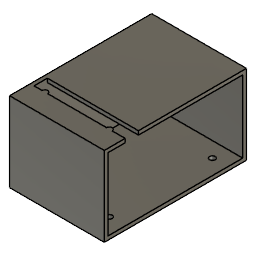
Tic housing (Autodesk Fusion 360 design; units mm, degrees)
Autodesk Fusion 360 part; units mm, degrees
sketch "Sketch1" plane through (0, 0, 0) normal (0, 0, 1) x (1, 0, 0)
  line L0 (-25, 50) -> (25, 50)
  line L1 (25, 50) -> (25, -25)
  line L2 (25, -25) -> (-25, -25)
  line L3 (-25, -25) -> (-25, 50)
  circle A0 centre (-17.3027, -14) radius 1.5
  circle A1 centre (16.6973, -14) radius 1.5
  circle A2 centre (-17, 40) radius 1.5
  circle A3 centre (17, 39.9992) radius 1.5
  dimension "d1" = 3
  dimension "d2" = 3
  dimension "d4" = 34
  dimension "d5" = 3
  dimension "d6" = 54
  dimension "d7" = 3
  dimension "d9" = 34
  dimension "d10" = 54
  constraint horizontal L0
  constraint vertical L1
  constraint horizontal L2
  constraint vertical L3
  measures "d1" diameter of A0
  measures "d2" diameter of A1
  measures "d4" horizontal distance of A0.centre A1.centre
  measures "d5" diameter of A2
  measures "d6" vertical distance of A0.centre A2.centre
  measures "d7" diameter of A3
  measures "d9" horizontal distance of A2.centre A3.centre
  measures "d10" distance of A1.centre A3.centre
extrude "Extrude1" add sketch "Sketch1" along normal blind 2 makes body 1
ref_plane "WorkPlane1" through (0, 12.5, 3) normal (0, 0, 1) x (1, 0, 0)
ref_plane "WorkPlane2" through (0, 12.5, 42) normal (0, 0, 1) x (1, 0, 0)
sketch "Sketch4" plane through (0, 0, 42) normal (0, 0, 1) x (1, 0, 0)
sketch "Sketch5" plane through (0, 0, 42) normal (0, 0, 1) x (1, 0, 0)
  line L0 (25, -25) -> (-25, -25)
  line L1 (-25, -25) -> (-25, 50)
  line L2 (-25, 50) -> (25, 50)
  line L3 (25, 50) -> (25, -25)
  constraint horizontal L0
  constraint vertical L1
  constraint horizontal L2
  constraint vertical L3
extrude "Extrude2" add sketch "Sketch5" against normal blind 2 separate body makes body 2
sketch "Sketch6" plane through (0, 0, 2) normal (0, 0, 1) x (-1, 0, 0)
  circle A0 centre (17, -40) radius 1.5
  circle A1 centre (-16.6973, 14) radius 1.5
  circle A2 centre (-17, -39.9992) radius 1.5
  circle A3 centre (17.3027, 14) radius 1.5
  line L0 (25, 25) -> (-25, 25)
  line L1 (-25, 25) -> (-25, -50)
  line L2 (-25, -50) -> (25, -50)
  line L3 (25, -50) -> (25, 25)
  line L4 (25, -50) -> (23, -50)
  line L5 (23, -50) -> (23, 25)
  line L6 (23, 25) -> (25, 25)
  line L7 (25, 25) -> (25, -50)
  constraint horizontal L4
  constraint vertical L5
  constraint horizontal L6
  constraint vertical L7
  constraint coincident L0 L5.end
  constraint coincident L2.end L3.start
extrude "Extrude3" add sketch "Sketch6" along normal blind 39 contours L0 L2 L3 L4 L5 L6 L7 bodies 1 2
sketch "Sketch7" plane through (0, 0, 2) normal (0, 0, 1) x (-1, 0, 0)
  line L0 (23, -50) -> (23, 25)
  line L1 (23, 25) -> (-25, 25)
  line L2 (-25, 25) -> (-25, -50)
  line L3 (-25, -50) -> (23, -50)
  circle A0 centre (17.3027, 14) radius 1.5
  circle A1 centre (-17, -39.9992) radius 1.5
  circle A2 centre (-16.6973, 14) radius 1.5
  circle A3 centre (17, -40) radius 1.5
  line L4 (23, 25) -> (-25, 25)
  line L5 (-25, 25) -> (-25, 23)
  line L6 (-25, 23) -> (23, 23)
  line L7 (23, 23) -> (23, 25)
  line L8 (23, -50) -> (-25, -50)
  line L9 (-25, -50) -> (-25, -48)
  line L10 (-25, -48) -> (23, -48)
  line L11 (23, -48) -> (23, -50)
  constraint horizontal L4
  constraint vertical L5
  constraint horizontal L6
  constraint vertical L7
  constraint coincident L2 L5.end
  constraint coincident L0.end L1.start
  constraint horizontal L8
  constraint vertical L9
  constraint horizontal L10
  constraint vertical L11
  constraint coincident L2 L9.end
  constraint coincident L0.start L3.end
extrude "Extrude4" add sketch "Sketch7" along normal blind 38 contours L0 L2 L3 L8 L9 L10 L11 bodies 1
extrude "Extrude5" add sketch "Sketch7" along normal blind 38 contours L0 L1 L2 L4 L5 L6 L7 bodies 1
sketch "Sketch8" plane through (0, 0, 2) normal (0, 0, 1) x (-1, 0, 0)
  line L0 (23, 23) -> (-25, 23)
  line L1 (-25, 23) -> (-25, -48)
  line L2 (-25, -48) -> (23, -48)
  line L3 (23, -48) -> (23, 23)
  circle A0 centre (17, -40) radius 1.5
  circle A1 centre (-16.6973, 14) radius 1.5
  circle A2 centre (-17, -39.9992) radius 1.5
  circle A3 centre (17.3027, 14) radius 1.5
  line L4 (23, 14) -> (-25, 14)
  line L5 (-25, 14) -> (-25, 7)
  line L6 (-25, 7) -> (23, 7)
  line L7 (23, 7) -> (23, 14)
  constraint horizontal L4
  constraint vertical L5
  constraint horizontal L6
  constraint vertical L7
  constraint coincident L1 L5.end
  constraint coincident L3 L4.start
extrude "Extrude6" cut sketch "Sketch8" along normal blind 48 contours L1 L3 A1 A3 L4 L5 L6 L7 bodies 1
